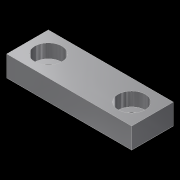
# Autodesk Inventor part: Part1
Saved by Autodesk Inventor 2021.1 (Build 251245000, 245)
## iProperties
Created: 2020-08-29
Part Number: Part1
Material: A5052
Document SubType Name: Modeling
Designer: Hashimoto
Mass: 4.06564 g
Surface Area: 10 cm^2
Volume: 1.5 cm^3
Density: 2.71043 g/cm^3
Appearance: アルミニウム - つや出し
Author: Hashimoto
Autodesk Inventor part; units mm, degrees
ref_plane "YZ Plane" through (0, 0, 0) normal (1, 0, 0) x (0, 1, 0)
ref_plane "XZ Plane" through (0, 0, 0) normal (0, 1, 0) x (-1, 0, 0)
ref_plane "XY Plane" through (0, 0, 0) normal (0, 0, 1) x (1, 0, 0)
sketch "スケッチ22" plane through (0, 0, 0) normal (0, 0, 1) x (1, 0, 0)
  line L0 (-15, -5) -> (-15, 5)
  line L1 (-15, 5) -> (15, 5)
  line L2 (15, 5) -> (15, -5)
  line L3 (15, -5) -> (-15, -5)
  point P0 (0, 0)
  point P1 (-15, 0)
  point P2 (0, -5)
  dimension "d144" = 10
  dimension "d145" = 30
  constraints: 8 end point, 2 midpoint, 2 perpendicular, 1 horizontal, 1 horizontal alignment, 1 vertical, 1 vertical alignment
  measures "d144" distance of L0.start L0.end
  measures "d145" distance of L2.end L0.start
extrude "押し出し14" add sketch "スケッチ22" along normal blind 5
sketch "スケッチ23" plane through (0, 0, 5) normal (0, 0, 1) x (1, 0, 0)
  point P0 (0, 0)
  point P1 (10, 0)
  point P2 (-10, 0)
  dimension "d146" = 20
  dimension "d147" = 10
  constraints: 2 horizontal alignment
  measures "d146" distance of point (10, 0) point (-10, 0)
  measures "d147" distance of point (0, 0) point (-10, 0)
hole "穴9" [suppressed]
equation "\"d147\" = 0.5 * d146"
